Autodesk Inventor part; units mm, degrees
(part 2 of 2)
sketch "Skizze14" plane through (0, 0, 0) normal (0, 0, 1) x (1, 0, 0)
  arc A0 (18, 44.9917) -> (0, 44.9917) centre (9, 60) ccw projected
  line L0 (-8.393, 58.0674) -> (31.5, 62.5) construction
  line L1 (31.5, 57.5) -> (-13.5, 62.5) construction
  line L2 (31.5, 57.5) -> (34, 60)
  line L3 (31.5, 57.5) -> (38.5711, 57.5) construction
  line L4 (31.5, 62.5) -> (34, 60)
  line L5 (31.5, 62.5) -> (37.2148, 62.5) construction
  line L6 (26.3205, 57.5) -> (31.5, 57.5)
  line L7 (31.5, 62.5) -> (26.3205, 62.5)
  arc A1 (26.3205, 57.5) -> (26.3205, 62.5) centre (9, 60) ccw
  arc A2 (-8.3205, 62.5) -> (-8.393, 61.9326) centre (9, 60) ccw
  arc A3 (-8.393, 58.0674) -> (-8.3205, 57.5) centre (9, 60) ccw
  point P0 (0, 0)
  constraints: 16 end point, 6 point on circle, 3 centre point, 3 horizontal, 2 point on line, 1 coincident, 1 midpoint, 1 parallel
extrude "Extrusion13" add sketch "Skizze14" along normal blind 2
sketch "Skizze15" plane through (0, 0, 2) normal (0, 0, 1) x (1, 0, 0)
  line L0 (34, 60) -> (31.5, 62.5) projected
  line L1 (31.5, 62.5) -> (26.3205, 62.5) projected
  arc A0 (26.3205, 57.5) -> (26.3205, 62.5) centre (9, 60) ccw projected
  line L2 (26.3205, 57.5) -> (31.5, 57.5) projected
  line L3 (31.5, 57.5) -> (34, 60) projected
  line L4 (33.3501, 59.3501) -> (26.4879, 59.3501)
  line L5 (26.4879, 60.6499) -> (33.3501, 60.6499)
  line L6 (42.7801, 60.6499) -> (42.7801, 59.3501)
  line L7 (31.5, 62.5) -> (34, 60) projected
  line L8 (42.7801, 59.3501) -> (26.4912, 60.5558) construction
  line L9 (26.4912, 59.4442) -> (42.7801, 60.6499) construction
  line L10 (33.3501, 60.6499) -> (34, 60)
  circle A1 centre (9, 60) radius 17.5
  line L11 (33.3501, 60.6499) -> (25.4991, 60.6499)
  line L12 (25.4991, 60.6499) -> (25.4991, 59.3708)
  line L13 (25.4991, 59.3708) -> (33.3501, 59.3708)
  line L14 (33.3501, 59.3708) -> (33.3501, 60.6499)
  point P0 (0, 0)
  constraints: 20 end point, 4 point on circle, 4 point on line, 3 parallel, 2 horizontal, 1 coincident, 1 collinear, 1 perpendicular, 3 other
extrude "Extrusion14" add sketch "Skizze15" along normal blind 2 contours L14 L13 A0 L5 | A0 L13 L12 L11
sketch "Skizze16" plane through (0, 0, 2) normal (0, 0, 1) x (1, 0, 0)
  line L0 (33.3501, 59.3708) -> (26.4887, 59.3708) projected
  arc A0 (26.3205, 57.5) -> (26.4887, 59.3708) centre (9, 60) ccw projected
  line L1 (26.3205, 57.5) -> (31.5, 57.5) projected
  line L2 (31.5, 57.5) -> (34, 60) projected
  line L3 (34, 60) -> (33.3501, 60.6499) projected
  line L4 (33.3501, 60.6499) -> (33.3501, 59.3708) projected
  line L5 (33.3501, 59.3708) -> (33.3501, 60.6499) projected
  line L6 (33.3501, 60.6499) -> (33.3501, 59.3708)
  line L7 (31.5, 57.5) -> (34, 60) projected
  line L8 (33.3501, 59.3708) -> (34, 60)
  line L9 (34, 60) -> (33.3501, 60.6499) projected
  line L10 (34, 60) -> (33.3501, 60.6499)
  point P0 (0, 0)
  constraints: 6 end point, 2 collinear
extrude "Extrusion15" add sketch "Skizze16" along normal blind 2 contours L4 L3 L8
sketch "Skizze17" plane through (26.4887, 59.3708, 2) normal (0, -1, 0) x (1, 0, 0)
  line L0 (7.5113, 2) -> (6.8614, 2) projected
  line L1 (7.5113, 2) -> (4.9631, 2)
  line L2 (0, 2) -> (6.8614, 2) projected
  line L3 (4.9631, 2) -> (7.5113, -0.0321)
  line L4 (7.5113, -0.0321) -> (7.5113, 2)
  point P0 (-26.4887, -2)
  constraints: 6 end point, 1 perpendicular, 1 point on line
extrude "Extrusion16" cut sketch "Skizze17" against normal through all
ref_plane "Arbeitsebene3" through (0, 0, 35) normal (0, 0, 1) x (1, 0, 0)
